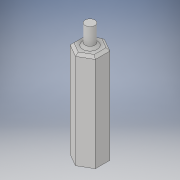
# Autodesk Inventor part: HexShaft1
Saved by Autodesk Inventor 2017 (Build 210142000, 142)
## iProperties
Created: 2017-10-26
Part Number: HexShaft1
Material: Generic
Document SubType Name: Modeling
Designer: Aidan_Moga
Density: 1 g/cm^3
Appearance: Default
Author: Aidan_Moga
Autodesk Inventor part; units mm, degrees
ref_plane "YZ Plane" through (0, 0, 0) normal (1, 0, 0) x (0, 1, 0)
ref_plane "XZ Plane" through (0, 0, 0) normal (0, 1, 0) x (-1, 0, 0)
sketch "Sketch1" plane through (0, 0, 0) normal (0, 1, 0) x (-1, 0, 0)
  line L0 (16.4978, 9.525) -> (16.4978, -9.525)
  line L1 (16.4978, -9.525) -> (0, -19.05)
  line L2 (0, -19.05) -> (-16.4978, -9.525)
  line L3 (-16.4978, 9.525) -> (-16.4978, -9.525)
  line L4 (-16.4978, 9.525) -> (0, 19.05)
  line L5 (0, 19.05) -> (16.4978, 9.525)
  circle A0 centre (0, 0) radius 19.05 construction
  line L6 (0, 25.4) -> (0, -25.4) construction
  circle A1 centre (0, 0) radius 6.35
  dimension "d0" = 38.1
  dimension "d8" = 12.7
  constraints: 14 end point, 6 point on circle, 3 equal length, 2 centre point, 2 parallel, 1 coincident, 1 point on line, 1 vertical
  measures "d0" diameter of A0
  measures "d8" diameter of A1
extrude "Hexagon1" add sketch "Sketch1" along normal blind 127 contours L0 L1 L2 L3 L4 L5 | A1
sketch "Sketch2" plane through (0, 127, 0) normal (0, 1, 0) x (1, 0, 0)
  circle A0 centre (0, 0) radius 6.35
  line L0 (0, 0) -> (25.4, 0) construction
  dimension "d3" = 12.7
  constraints: 2 end point, 1 centre point, 1 coincident, 1 horizontal
  measures "d3" diameter of A0
ref_plane "Work Plane2" through (0, 127, 0) normal (1, 0, 0) x (0, 0, -1)
sketch "Sketch5" plane through (0, 127, 0) normal (1, 0, 0) x (0, 0, -1)
  line L0 (9.525, 0) -> (-9.525, 0) projected
  line L1 (0, 0) -> (0, 25.4)
  point P0 (0, -127)
  dimension "d9" = 25.4
  constraints: 2 end point, 1 midpoint, 1 vertical
  measures "d9" distance of L1.start L1.end
sweep "Sweep1" add profiles "Sketch2" path "Sketch5" path curves L1
chamfer "Chamfer1" distance 3.175 angle 45 7 edges at (8.2489, 127, -14.2875) (-6.35, 127, 0) (16.4978, 127, 0) (8.2489, 127, 14.2875) (-8.2489, 127, -14.2875) (-16.4978, 127, 0) (-8.2489, 127, 14.2875)
body "Solid1"
